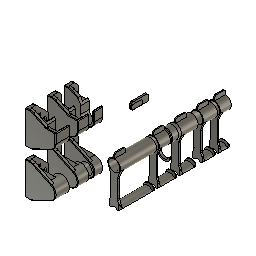
SKADIS_SNS_TapeStorage (Autodesk Fusion 360 design; units mm, degrees)
Autodesk Fusion 360 part; units mm, degrees
(part 1 of 2)
sketch "SlotLayout" plane through (0, 0, 0) normal (1, 0, 0) x (0, 1, 0)
  line L0 (-22.4, 25) -> (-22.4, 15)
  line L1 (82.4, 5) -> (82.4, -5)
  line L2 (-37.6, -5) -> (-37.6, 5)
  line L3 (-80, 5) -> (-80, -5) construction
  line L4 (-97.6, 15) -> (-97.6, 25)
  line L5 (2.4, -5) -> (2.4, 5)
  arc A0 (-77.6, 5) -> (-82.4, 5) centre (-80, 5) ccw
  arc A1 (22.4, 25) -> (17.6, 25) centre (20, 25) ccw
  arc A2 (-97.6, 25) -> (-102.4, 25) centre (-100, 25) ccw
  arc A3 (97.6, 15) -> (102.4, 15) centre (100, 15) ccw
  line L6 (-60, 25) -> (-60, 15) construction
  line L7 (-77.6, -5) -> (-77.6, 5)
  arc A4 (77.6, -5) -> (82.4, -5) centre (80, -5) ccw
  line L8 (-40, 5) -> (-40, -5) construction
  line L9 (-57.6, 15) -> (-57.6, 25)
  line L10 (-62.4, 25) -> (-62.4, 15)
  line L11 (-102.4, 25) -> (-102.4, 15)
  line L12 (97.6, 15) -> (97.6, 25)
  arc A5 (-102.4, 15) -> (-97.6, 15) centre (-100, 15) ccw
  line L13 (20, 25) -> (20, 15) construction
  line L14 (22.4, 25) -> (22.4, 15)
  line L15 (-80, 0) -> (0, 0) construction
  line L16 (62.4, 25) -> (62.4, 15)
  line L17 (42.4, 5) -> (42.4, -5)
  arc A6 (2.5, 5) -> (-2.5, 5) centre (0, 5) ccw
  arc A7 (2.4, 5) -> (-2.4, 5) centre (0, 5) ccw
  line L18 (80, 5) -> (80, -5) construction
  arc A8 (82.4, 5) -> (77.6, 5) centre (80, 5) ccw
  arc A9 (-2.5, -5) -> (2.5, -5) centre (0, -5) ccw
  arc A10 (57.6, 15) -> (62.4, 15) centre (60, 15) ccw
  arc A11 (62.4, 25) -> (57.6, 25) centre (60, 25) ccw
  line L19 (17.6, 15) -> (17.6, 25)
  line L20 (-20, 25) -> (-20, 15) construction
  line L21 (-42.4, 5) -> (-42.4, -5)
  line L22 (60, 25) -> (60, 15) construction
  arc A12 (42.4, 5) -> (37.6, 5) centre (40, 5) ccw
  line L23 (-100, 25) -> (-100, 15) construction
  line L24 (100, 25) -> (100, 15) construction
  arc A13 (-57.6, 25) -> (-62.4, 25) centre (-60, 25) ccw
  arc A14 (37.6, -5) -> (42.4, -5) centre (40, -5) ccw
  line L25 (40, 5) -> (40, -5) construction
  line L26 (-17.6, 15) -> (-17.6, 25)
  arc A15 (-17.6, 25) -> (-22.4, 25) centre (-20, 25) ccw
  line L27 (-82.4, 5) -> (-82.4, -5)
  line L28 (-2.5, 5) -> (-2.5, -5)
  line L29 (-2.4, 5) -> (-2.4, -5)
  line L30 (102.4, 25) -> (102.4, 15)
  arc A16 (17.6, 15) -> (22.4, 15) centre (20, 15) ccw
  arc A17 (-22.4, 15) -> (-17.6, 15) centre (-20, 15) ccw
  line L31 (37.6, -5) -> (37.6, 5)
  line L32 (0, 5) -> (0, -5) construction
  arc A18 (-62.4, 15) -> (-57.6, 15) centre (-60, 15) ccw
  arc A19 (-42.4, -5) -> (-37.6, -5) centre (-40, -5) ccw
  arc A20 (-2.4, -5) -> (2.4, -5) centre (0, -5) ccw
  arc A21 (102.4, 25) -> (97.6, 25) centre (100, 25) ccw
  arc A22 (-82.4, -5) -> (-77.6, -5) centre (-80, -5) ccw
  arc A23 (-37.6, 5) -> (-42.4, 5) centre (-40, 5) ccw
  line L33 (77.6, -5) -> (77.6, 5)
  line L34 (57.6, 15) -> (57.6, 25)
  line L35 (2.5, -5) -> (2.5, 5)
  arc A24 (22.4, -15) -> (17.6, -15) centre (20, -15) ccw
  line L36 (17.6, -15) -> (17.6, -25)
  arc A25 (17.6, -25) -> (22.4, -25) centre (20, -25) ccw
  line L37 (22.4, -25) -> (22.4, -15)
  line L38 (-22.4, -25) -> (-22.4, -15)
  arc A26 (-17.6, -15) -> (-22.4, -15) centre (-20, -15) ccw
  arc A27 (-22.4, -25) -> (-17.6, -25) centre (-20, -25) ccw
  line L39 (-17.6, -15) -> (-17.6, -25)
  line L40 (-62.4, -25) -> (-62.4, -15)
  arc A28 (-57.6, -15) -> (-62.4, -15) centre (-60, -15) ccw
  arc A29 (-62.4, -25) -> (-57.6, -25) centre (-60, -25) ccw
  line L41 (-57.6, -15) -> (-57.6, -25)
  arc A30 (57.6, -25) -> (62.4, -25) centre (60, -25) ccw
  line L42 (62.4, -25) -> (62.4, -15)
  arc A31 (62.4, -15) -> (57.6, -15) centre (60, -15) ccw
  line L43 (57.6, -15) -> (57.6, -25)
  point P0 (-20, 20)
  point P1 (-40, 0)
  dimension "d179_1_1_1" = 0
  dimension "d181_1_1_1" = 0
  dimension "d187_1_1_1" = 10
  constraint tangent L27 A22
  constraint tangent L7 A22
  constraint parallel L7 L27
  constraint tangent A0 L7
  constraint tangent A0 L27
  constraint vertical L3
  constraint tangent L21 A19
  constraint tangent L2 A19
  constraint parallel L2 L21
  constraint tangent L2 A23
  constraint tangent L21 A23
  constraint vertical L8
  constraint tangent L29 A20
  constraint tangent L5 A20
  constraint parallel L5 L29
  constraint tangent L5 A7
  constraint tangent A7 L29
  constraint parallel L2 L32
  constraint midpoint L15.start L3
  constraint midpoint L15.end L32
  constraint horizontal L15
  constraint equal L8 L32
  constraint equal L3 L8
  constraint midpoint P1 L8
  constraint coincident P1 L15
  constraint equal A7 A23
  constraint equal A0 A23
  constraint coincident L15.end origin
  constraint symmetric A0.end L1.start L32
  constraint symmetric L1.end L27.end L32
  constraint symmetric L7.start A4.start L32
  constraint symmetric A8.end A0.start L32
  constraint symmetric A4 L32 A22
  constraint symmetric A0 A8 L32
  constraint symmetric L17.start L21.start L32
  constraint symmetric L17.end L21.end L32
  constraint symmetric A14.start L2.start L32
  constraint symmetric A12.end L2.end L32
  constraint symmetric A14 L32 A19
  constraint symmetric A12 L32 A23
  constraint tangent L0 A17
  constraint tangent L26 A17
  constraint parallel L0 L26
  constraint tangent L26 A15
  constraint tangent L0 A15
  constraint vertical L20
  constraint equal L20 L32
  constraint equal A7 A15
  constraint midpoint P0 L20
  constraint symmetric L0.end L14.end L32
  constraint symmetric L26.end A1.end L32
  constraint symmetric L0.start A1.start L32
  constraint symmetric L26.start L19.start L32
  constraint symmetric A1 A15 L32
  constraint symmetric A16 A17 L32
  constraint symmetric A11.end L9.end L32
  constraint symmetric L16.start L10.start L32
  constraint symmetric A11 A13 L32
  constraint symmetric L16.end L10.end L32
  constraint symmetric A10.start L9.start L32
  constraint symmetric A10 L32 A18
  constraint symmetric L12.end L4.end L32
  constraint symmetric L30.start A2.end L32
  constraint symmetric A2 L32 A21
  constraint symmetric A3.end L11.end L32
  constraint symmetric A3.start L4.start L32
  constraint symmetric A3 A5 L32
  constraint symmetric L0.start L15 L38.start
  constraint symmetric L0.end L15 L38.end
  constraint symmetric A10.start L15 A31.end
  constraint symmetric L16.end L15 L42.end
  constraint symmetric L26.start L15 A26.start
  constraint symmetric L26.end L15 A27.end
  constraint symmetric L19.start L15 A24.end
  constraint symmetric A11.end L15 A30.start
  constraint symmetric L14.end L15 A24.start
  constraint symmetric A1.end L15 L36.end
  constraint symmetric A1.start L15 A25.end
  constraint symmetric L16.start L15 A30.end
  constraint symmetric L10.end L15 L40.end
  constraint symmetric L9.start L15 A28.start
  constraint symmetric L9.end L15 A29.end
  constraint symmetric L10.start L15 L40.start
  constraint symmetric A1 L15 A25
  constraint symmetric L15 A10 A31
  constraint symmetric L15 A11 A30
  constraint symmetric L15 A13 A29
  constraint symmetric L15 A15 A27
  constraint symmetric L15 A16 A24
  constraint symmetric L15 A17 A26
  constraint symmetric L15 A18 A28
  measures "d22" distance of A6.centre A9.centre
  measures "d23" radius of A7
  measures "d4" distance of L8 L32
  measures "d25" distance of L3 L8
  measures "d26" distance of L20.end A6.centre
  measures "d27" distance of P0 L15.end
  measures "d107" radius of A3.end
sketch "PrintKey" plane through (0, 0, 0) normal (1, 0, 0) x (0, 1, 0)
  circle A0 centre (0, 0) radius 1.6
  line L0 (2.6, -6.7) -> (-2.6, -6.7)
  line L1 (-2.6, -6.7) -> (-2.6, 6.7)
  line L2 (-2.6, 6.7) -> (2.6, 6.7)
  line L3 (2.6, 6.7) -> (2.6, -6.7)
  line L4 (0, 6.7) -> (0, -6.7) construction
  line L5 (0, 6.7) -> (0, 23.5939) construction
  line L6 (0, 23.5939) -> (-8.4469, 15.1469) construction
  line L7 (-8.4469, 15.1469) -> (8.4469, 15.1469) construction
  line L8 (8.4469, 15.1469) -> (0, 23.5939) construction
  circle A1 centre (0, 0) radius 3.4
  line L9 (17.4, -6.7) -> (17.4, 6.7)
  line L10 (22.6, -6.7) -> (17.4, -6.7)
  line L11 (22.6, 6.7) -> (22.6, -6.7)
  line L12 (17.4, 6.7) -> (22.6, 6.7)
  circle A2 centre (20, 0) radius 1.6
  circle A3 centre (20, 0) radius 3.4
  line L13 (20, 6.7) -> (20, -6.7) construction
  line L14 (37.4, -6.7) -> (37.4, 6.7)
  line L15 (42.6, -6.7) -> (37.4, -6.7)
  line L16 (42.6, 6.7) -> (42.6, -6.7)
  line L17 (37.4, 6.7) -> (42.6, 6.7)
  circle A4 centre (40, 0) radius 1.6
  circle A5 centre (40, 0) radius 3.4
  line L18 (40, 6.7) -> (40, -6.7) construction
  line L19 (57.4, -6.7) -> (57.4, 6.7)
  line L20 (62.6, -6.7) -> (57.4, -6.7)
  line L21 (62.6, 6.7) -> (62.6, -6.7)
  line L22 (57.4, 6.7) -> (62.6, 6.7)
  circle A6 centre (60, 0) radius 1.6
  circle A7 centre (60, 0) radius 3.4
  line L23 (60, 6.7) -> (60, -6.7) construction
  line L24 (-22.6, -6.7) -> (-22.6, 6.7)
  line L25 (-22.6, 6.7) -> (-17.4, 6.7)
  line L26 (-17.4, -6.7) -> (-22.6, -6.7)
  line L27 (-17.4, 6.7) -> (-17.4, -6.7)
  line L28 (-20, 6.7) -> (-20, -6.7) construction
  circle A8 centre (-20, 0) radius 3.4
  circle A9 centre (-20, 0) radius 1.6
  line L29 (-42.6, -6.7) -> (-42.6, 6.7)
  line L30 (-42.6, 6.7) -> (-37.4, 6.7)
  line L31 (-37.4, -6.7) -> (-42.6, -6.7)
  line L32 (-37.4, 6.7) -> (-37.4, -6.7)
  line L33 (-40, 6.7) -> (-40, -6.7) construction
  circle A10 centre (-40, 0) radius 3.4
  circle A11 centre (-40, 0) radius 1.6
  line L34 (-62.6, -6.7) -> (-62.6, 6.7)
  line L35 (-62.6, 6.7) -> (-57.4, 6.7)
  line L36 (-57.4, -6.7) -> (-62.6, -6.7)
  line L37 (-57.4, 6.7) -> (-57.4, -6.7)
  line L38 (-60, 6.7) -> (-60, -6.7) construction
  circle A12 centre (-60, 0) radius 3.4
  circle A13 centre (-60, 0) radius 1.6
  line L39 (-22.6, 13.3) -> (-22.6, 26.7)
  line L40 (-22.6, 26.7) -> (-17.4, 26.7)
  line L41 (-17.4, 26.7) -> (-17.4, 13.3)
  line L42 (-17.4, 13.3) -> (-22.6, 13.3)
  line L43 (-20, 26.7) -> (-20, 13.3) construction
  circle A14 centre (-20, 20) radius 3.4
  circle A15 centre (-20, 20) radius 1.6
  line L44 (0, 0) -> (-32.4518, 0) construction
  line L45 (-22.6, -26.7) -> (-17.4, -26.7)
  circle A16 centre (-20, -20) radius 1.6
  line L46 (-22.6, -13.3) -> (-22.6, -26.7)
  circle A17 centre (-20, -20) radius 3.4
  line L47 (-20, -26.7) -> (-20, -13.3) construction
  line L48 (-17.4, -26.7) -> (-17.4, -13.3)
  line L49 (-17.4, -13.3) -> (-22.6, -13.3)
  point P0 (20, 0)
  point P1 (20, 0)
  point P2 (20, 0)
  point P3 (40, 0)
  point P4 (40, 0)
  point P5 (40, 0)
  point P6 (60, 0)
  point P7 (60, 0)
  point P8 (60, 0)
  dimension "d21" = 13.4
  dimension "d24" = 5.2
  dimension "d28" = 3.2
  dimension "d34" = 6.8
  dimension "d37" = 20
  dimension "d38" = 0
  dimension "d41" = -20
  dimension "d42" = 0
  dimension "d151" = 0
  dimension "d152" = 20
  constraint horizontal L2
  constraint vertical L3
  constraint horizontal L0
  constraint vertical L1
  constraint midpoint L4.start L2
  constraint midpoint L4.end L0
  constraint midpoint A0.centre L4
  constraint coincident A0.centre A1.centre
  constraint perpendicular L2 L5
  constraint perpendicular L5 L7
  constraint midpoint L5 L7
  constraint perpendicular L6 L8
  constraint perpendicular L28 L44
  constraint symmetric L39.start L44 L46.start
  constraint symmetric L39.end L44 L45.start
  constraint symmetric L40.end L44 L45.end
  constraint symmetric L41.end L44 L48.end
  constraint symmetric L43.start L44 L47.start
  constraint symmetric L43.end L44 L47.end
  constraint symmetric A14 L44 A17
  constraint symmetric A15 L44 A16
  measures "d21" distance of L4.end L4.start
  measures "d24" distance of L1 L3
  measures "d28" diameter of A0
  measures "d34" diameter of A1
sketch "Hanger_Profile" plane through (0, 0, 0) normal (0, 1, 0) x (1, 0, 0)
  line L0 (0, 0) -> (60, 0) construction
  circle A0 centre (60, 0) radius 10.2
  circle A1 centre (60, 0) radius 11.4
  line L1 (60, 0) -> (60, 71.4) construction
  arc A2 (51.3397, 62.3861) -> (68.6603, 62.3861) centre (60, 71.4) ccw
  arc A3 (51.3397, 66.4) -> (68.6603, 66.4) centre (60, 71.4) ccw
  line L2 (51.3397, 66.4) -> (51.3397, 58.4)
  line L3 (51.3397, 58.4) -> (54, 51.091)
  line L4 (54, 51.091) -> (54, 9.6933)
  line L5 (51.3397, 66.4) -> (60, 71.4)
  line L6 (60, 71.4) -> (68.6603, 66.4)
  line L7 (68.6603, 66.4) -> (68.6603, 58.4)
  line L8 (68.6603, 58.4) -> (66, 51.091)
  line L9 (66, 51.091) -> (66, 9.6933)
  circle A4 centre (60, 0) radius 10
  line L10 (59, -11.3561) -> (59, -19.3561)
  line L11 (59, -19.3561) -> (61, -19.3561)
  line L12 (61, -19.3561) -> (61, -11.3561)
  line L13 (60, 0) -> (60, -19.3561) construction
  line L14 (49.333, 4.0218) -> (54, 16.4)
  line L15 (70.667, 4.0218) -> (66, 16.4)
  arc A5 (53.9378, 67.9) -> (66.0622, 67.9) centre (60, 71.4) ccw
  point P0 (60, 11.4)
  point P1 (60, 61.4)
  point P2 (60, 58.9)
  dimension "d53" = 1.2
  dimension "d58" = 2.5
  dimension "d60" = 50
  dimension "d62" = 8
  dimension "d64" = 20
  dimension "d65" = 60
  dimension "d66" = 6
  dimension "d93" = 0.2
  dimension "d94" = 2
  dimension "d95" = 8
  dimension "d97" = 20
  dimension "d107" = 12.5
  dimension "d125" = 5
  dimension "d132" = 60
  dimension "d213" = 3
  constraint coincident L0.start origin
  constraint horizontal L0
  constraint coincident L0.end A0.centre
  constraint concentric A0 A1
  constraint perpendicular L0 L1
  constraint coincident A1 P0
  constraint coincident L1 P0
  constraint coincident P1 A3
  constraint coincident L1 P1
  constraint coincident L1.end A2.centre
  constraint coincident A1 L4.end
  constraint parallel L1 L4
  constraint concentric A2 A3
  constraint coincident L5 A3.start
  constraint parallel L1 L2
  constraint parallel L2 L7
  constraint horizontal L2.end L7.end
  constraint horizontal L3.end L8.end
  constraint parallel L4 L9
  constraint horizontal L4.end L9.end
  constraint coincident A1 L9.end
  constraint concentric A0 A4
  constraint coincident A1 L10.start
  constraint vertical L10
  constraint perpendicular L10 L11
  constraint coincident A1 L12.end
  constraint perpendicular L11 L12
  constraint midpoint L11 L13.end
  constraint vertical L13
  constraint coincident L7 A2.end
  constraint coincident A2 P2
  constraint coincident L2 A2.start
  constraint vertical P1 P2
  constraint horizontal A3.start A3.end
  constraint coincident A1 L14.start
  constraint coincident L4 L14.end
  constraint coincident A1 L15.start
  constraint coincident L9 L15.end
  constraint horizontal L14.end L15.end
  constraint tangent A1 L14
  constraint tangent A1 L15
  constraint coincident L5 A5.start
  constraint horizontal A5.start A5.end
  measures "d53" distance of A0 A1
  measures "d58" distance of P1 P2
  measures "d60" distance of P0 P1
  measures "d62" distance of L2.end A3.start
  measures "d64" angle of L3 L4
  measures "d65" angle of L1 L5
  measures "d66" distance of L1 L4
  measures "d93" distance of A0 A4
  measures "d94" distance of L10.end L11.end
  measures "d95" vertical distance of L12.end L13.end
  measures "d97" diameter of A4
  measures "d107" radius of A2
  measures "d125" vertical distance of P0 L14.end
  measures "d132" distance of L0.start L0.end
  measures "d213" distance of A3.start A5.start
sketch "SideBracket_SideProfile" plane through (0, 0, 0) normal (0, 1, 0) x (1, 0, 0)
  line L0 (0, -30) -> (0, 30)
  arc A0 (40, -14.1) -> (46.09, 12.717) centre (40, 0) ccw
  line L1 (46.09, 12.717) -> (10, 30)
  line L2 (10, 30) -> (0, 30)
  circle A1 centre (40, 0) radius 10.1
  circle A2 centre (40, 0) radius 14.1
  line L3 (10, -30) -> (46.09, -12.717)
  line L4 (5, 30) -> (5, -30)
  line L5 (40, 14.1) -> (5, 14.1)
  line L6 (5, 10.1) -> (49.8387, 10.1)
  line L7 (40, -14.1) -> (5, -14.1)
  line L8 (5, -10.1) -> (49.8387, -10.1)
  line L9 (0, -30) -> (10, -30)
  line L10 (50.1, 0) -> (50.1, -13.5)
  line L11 (54.1, -15.75) -> (54.1, 0)
  line L12 (29.9, 0) -> (29.9, -13.5)
  line L13 (25.9, 0) -> (25.9, -15.75)
  line L14 (52.1207, -17) -> (50.1, -13.5)
  line L15 (52.85, -17) -> (27.15, -17)
  arc A3 (52.85, -17) -> (54.1, -15.75) centre (52.85, -15.75) ccw
  arc A4 (25.9, -15.75) -> (27.15, -17) centre (27.15, -15.75) ccw
  line L16 (27.8793, -17) -> (29.9, -13.5)
  line L17 (27.8793, -17) -> (24.338, -23.1338)
  point P0 (60, 0)
  dimension "d133" = 30
  dimension "d134" = 30
  dimension "d136" = 40
  dimension "d137" = 20.2
  dimension "d140" = 4
  dimension "d174" = 5
  dimension "d175" = 10
  dimension "d178" = 4
  dimension "d182" = 4
  dimension "d183" = 10
  dimension "d184" = 30
  dimension "d258" = 30
  dimension "d259" = 2.5
  dimension "d260" = 17
  dimension "d261" = 30
  dimension "d262" = 3.5
  constraint vertical L0
  constraint coincident L0 origin
  constraint perpendicular L0 L2
  constraint concentric A0 A1
  constraint tangent A0 L1
  constraint concentric A1 A2
  constraint coincident A0.start A2
  constraint coincident A2 L3.end
  constraint tangent A0 L3
  constraint coincident L2 L4.start
  constraint coincident A2 L5.start
  constraint coincident L4 L5.end
  constraint perpendicular L4 L5
  constraint tangent A2 L5
  constraint coincident L4 L6.start
  constraint coincident A2 L6.end
  constraint perpendicular L4 L6
  constraint coincident L4 L7.end
  constraint tangent A2 L7
  constraint perpendicular L4 L7
  constraint coincident L4 L8.start
  constraint coincident A2 L8.end
  constraint perpendicular L4 L8
  constraint perpendicular L0 L9
  constraint coincident A1 L10.start
  constraint vertical L10
  constraint coincident A0 L11.end
  constraint vertical L11
  constraint tangent A1 L10
  constraint coincident A1 L12.start
  constraint coincident A2 L13.start
  constraint perpendicular L8 L13
  constraint tangent A2 L13
  constraint tangent A1 L12
  constraint horizontal L10.end L12.end
  constraint tangent L11 A3
  constraint tangent L13 A4
  constraint equal A3 A4
  constraint tangent L15 A4
  constraint perpendicular L13 L15
  constraint vertical L12
  constraint coincident L15 L14.start
  constraint coincident L15 L16.start
  constraint tangent L15 A3
  constraint tangent A2 L11
  constraint coincident L3 L17.end
  constraint parallel L16 L17
  measures "d133" distance of L0.start origin
  measures "d134" distance of L0.end origin
  measures "d136" distance of L0 A0.centre
  measures "d137" diameter of A1
  measures "d140" distance of A0 A1
  measures "d174" distance of L0 L4
  measures "d175" distance of L0.end L1.end
  measures "d178" distance of L5 L6
  measures "d182" distance of L7 L8
  measures "d183" distance of L0.start L3.start
  measures "d184" vertical distance of L0.start A0.centre
  measures "d258" angle of L11 L14
  measures "d259" diameter of A3
  measures "d260" distance of origin L15
  measures "d261" angle of L12 L16
  measures "d262" distance of L10.end L15
sketch "SideBracket_FrontProfile" plane through (0, 0, 0) normal (1, 0, 0) x (0, 1, 0)
  line L0 (-22.4, 25) -> (-22.4, 15) construction
  arc A0 (-22.4, 15) -> (-17.6, 15) centre (-20, 15) ccw construction
  line L1 (-17.6, 15) -> (-17.6, 25) construction
  arc A1 (-17.6, 25) -> (-22.4, 25) centre (-20, 25) ccw construction
  line L2 (2.5, -5) -> (2.5, 5) construction
  arc A2 (2.5, 5) -> (-2.5, 5) centre (0, 5) ccw construction
  arc A3 (-2.5, -5) -> (2.5, -5) centre (0, -5) ccw construction
  line L3 (-2.5, 5) -> (-2.5, -5) construction
  arc A4 (-22.4, -25) -> (-17.6, -25) centre (-20, -25) ccw construction
  line L4 (-22.4, -25) -> (-22.4, -15) construction
  arc A5 (-17.6, -15) -> (-22.4, -15) centre (-20, -15) ccw construction
  line L5 (-17.6, -15) -> (-17.6, -25) construction
  line L6 (-30, 30) -> (-30, 0)
  line L7 (-30, 0) -> (6, 0)
  line L8 (-30, 30) -> (-16, 30)
  line L9 (-16, 30) -> (6, 8)
  line L10 (6, 8) -> (6, 0)
  line L11 (-24, 30) -> (-24, 0)
  line L12 (-24, -30) -> (-24, 0)
  line L13 (-30, -30) -> (-16, -30)
  line L14 (-16, -30) -> (6, -8)
  line L15 (6, -8) -> (6, 0)
  line L16 (-30, -30) -> (-30, 0)
  line L17 (-16, 30) -> (-16, -30)
  line L18 (-10, 30) -> (-10, -30)
  line L19 (-10, -30) -> (-16, -30)
  line L20 (-16, 30) -> (-10, 30)
  point P0 (-20, 20)
  dimension "d145" = 6
  dimension "d146" = 10
  dimension "d148" = 3
  dimension "d153" = 4
  dimension "d154" = 6
  dimension "d159" = 5
  dimension "d198" = 10
  constraint parallel L1 L6
  constraint horizontal L7
  constraint coincident origin L7
  constraint perpendicular L6 L8
  constraint perpendicular L7 L10
  constraint coincident L8 L11.start
  constraint coincident L7 L11.end
  constraint perpendicular L7 L11
  constraint symmetric L6.start L7 L13.start
  constraint symmetric L6.end L7 L16.end
  constraint symmetric L10.end L7 L15.end
  constraint symmetric L7 L8.end L13.end
  constraint symmetric L7 L9.end L14.end
  constraint symmetric L7 L11.start L12.start
  constraint symmetric L7 L11.end L12.end
  constraint vertical L18
  constraint perpendicular L17 L20
  constraint perpendicular L18 L19
  measures "d145" distance of origin L7.end
  measures "d146" distance of P0 L6
  measures "d148" vertical distance of A2.centre L9.end
  measures "d153" horizontal distance of A1.centre L8.end
  measures "d154" distance of L6 L11
  measures "d159" distance of A1.centre L8
  measures "d198" distance of P0 L18
extrude "Extrude2" add sketch "SideBracket_FrontProfile" along normal blind 5 contours L6 L7 L8 L11 | L7 L12 L13 L16 | L7 L8 L11 L17 | L7 L12 L13 L17 | L7 L9 L17 L18 | L7 L14 L17 L18 | L7 L9 L10 L18 | L7 L14 L15 L18 makes body 1 in component "SideBracket_Heavy_"
extrude "Extrude1" add sketch "SideBracket_SideProfile" along normal blind 5 from surface at -30 contours L0 L2 L4 L9 | L3 L4 L7 L9 L13 L15 A4 L17 | L1 L2 A2 L4 L5 | L4 L7 L8 L13 | A2 L4 L5 L6 | A2 L4 L6 L8 L13 | L7 L8 L12 L13 L16 | L7 L13 L15 A4 L16 | L3 L15 L17 | A0 A2 L6 | A2 L8 L12 L13 | A2 L7 L8 L12 L16 | A0 A2 L3 L7 L15 L16 | A0 A1 A2 L6 L10 | A1 A2 L6 L12 | A2 L8 L12 | A0 A2 L8 | A1 | A1 A2 L8 L12 | A0 A1 A2 L8 L10 bodies 1 in component "SideBracket_Heavy_"
extrude "Extrude3" cut sketch "PrintKey" along normal blind 1.2 contours A0 | L0 L1 L3 A1 | L1 L3 A1 | L1 L2 L3 A1 | L39 L41 L42 A14 | L39 L41 A14 | L39 L40 L41 A14 | A15 | L45 L46 A17 L48 | L46 A17 L48 | L46 A17 L48 L49 | A16 bodies 1 in component "SideBracket_Heavy_"
extrude "Extrude6" add sketch "SideBracket_SideProfile" along normal blind 10 from surface at -25 contours L4 L7 L8 L13 | A2 L4 L5 L6 | L7 L8 L12 L13 L16 | A0 A2 L6 | A2 L7 L8 L12 L16 | A0 A1 A2 L6 L10 | A1 A2 L6 L12 | A0 A2 L8 | A1 A2 L8 L12 | A0 A1 A2 L8 L10 bodies 1 in component "SideBracket_Heavy_"
extrude "Extrude7" add sketch "SideBracket_SideProfile" along normal blind 10 from surface at -15 contours A0 A2 L6 | A0 A1 A2 L6 L10 | A1 A2 L6 L12 | A0 A2 L8 | A1 A2 L8 L12 | A0 A1 A2 L8 L10 bodies 1 in component "SideBracket_Heavy_"
chamfer "Chamfer3" distance 6 angle 45 2 edges at (5, -15, 12.1) (5, -15, -12.1) on bodies 1 in component "SideBracket_Heavy_"
extrude "Extrude4" cut sketch "PrintKey" along normal up to surface (5 mm away) contours A0 | A15 | A16 bodies 1 in component "SideBracket_Heavy_"
extrude "Extrude5" cut sketch "PrintKey" along normal up to surface (2.2 mm away) from surface at 2.8 contours L1 L3 A1 | L3 A1 | L1 A1 | L39 A14 | L39 L41 A14 | L41 A14 | L46 A17 | L46 A17 L48 | A17 L48 bodies 1 in component "SideBracket_Heavy_"
chamfer "Chamfer1" distance 1.8 angle 45 3 edges at (2.8, -23.1699, 18.7705) (2.8, -3.1699, -1.2295) (2.8, -23.1699, -21.2295) on bodies 1 in component "SideBracket_Heavy_"
fillet "Fillet1" radius 4 4 edges at (2.5, -16, 30) (2.5, 6, 8) (2.5, 6, -8) (2.5, -16, -30) on bodies 1 in component "SideBracket_Heavy_"
fillet "Fillet1" radius 16 2 edges at (10, -27.5, -30) (10, -27.5, 30) on bodies 1 in component "SideBracket_Heavy_"
fillet "Fillet1" radius 4 4 edges at (11, -15, 12.1) (11, -15, -12.1) (5, -9, -12.1) (5, -9, 12.1) on bodies 1 in component "SideBracket_Heavy_"
chamfer "Chamfer4" distance 1 angle 45 7 edges at (54.1, -30, 0) (29.6836, -30, 20.5738) (9.9098, -30, 29.6027) (3.1832, -30, 30) (3.1832, -30, -30) (9.9098, -30, -29.6027) (29.6836, -30, -20.5738) on bodies 1 in component "SideBracket_Heavy_"
extrude "Extrude2'" add sketch "SideBracket_FrontProfile" along normal blind 5 separate body contours L6 L7 L8 L11 | L7 L12 L13 L16 | L7 L8 L11 L17 | L7 L12 L13 L17 | L7 L9 L17 L18 | L7 L14 L17 L18 makes body 2 in component "SupportBracket_"
extrude "Extrude1'" add sketch "SideBracket_SideProfile" along normal blind 5 from surface at -30 contours L0 L2 L4 L9 | L3 L4 L7 L9 L13 L15 A4 L17 | L1 L2 A2 L4 L5 | L4 L7 L8 L13 | A2 L4 L5 L6 | A2 L4 L6 L8 L13 | L7 L8 L12 L13 L16 | L7 L13 L15 A4 L16 | L3 L15 L17 | A0 A2 L6 | A2 L8 L12 L13 | A2 L7 L8 L12 L16 | A0 A2 L3 L7 L15 L16 | A0 A1 A2 L6 L10 | A1 A2 L6 L12 | A2 L8 L12 | A0 A2 L8 | A1 A2 L8 L12 | A0 A1 A2 L8 L10 bodies 2 in component "SupportBracket_"
extrude "Extrude3'" cut sketch "PrintKey" along normal blind 1.2 contours A0 | L0 L1 L3 A1 | L1 L3 A1 | L1 L2 L3 A1 | L39 L41 L42 A14 | L39 L41 A14 | L39 L40 L41 A14 | A15 | L45 L46 A17 L48 | L46 A17 L48 | L46 A17 L48 L49 | A16 bodies 2 in component "SupportBracket_"
extrude "Extrude6'" add sketch "SideBracket_SideProfile" along normal blind 10 from surface at -25 contours L4 L7 L8 L13 | A2 L4 L5 L6 | L7 L8 L12 L13 L16 | A0 A2 L6 | A2 L7 L8 L12 L16 | A0 A1 A2 L6 L10 | A1 A2 L6 L12 | A0 A2 L8 | A1 A2 L8 L12 | A0 A1 A2 L8 L10 bodies 2 in component "SupportBracket_"
chamfer "Chamfer3'" distance 5 angle 45 2 edges at (5, -15, 12.1) (5, -15, -12.1) on bodies 2 in component "SupportBracket_"
extrude "Extrude4'" cut sketch "PrintKey" along normal up to surface (5 mm away) contours A0 | A15 | A16 bodies 2 in component "SupportBracket_"
extrude "Extrude5'" cut sketch "PrintKey" along normal up to surface (2.2 mm away) from surface at 2.8 contours L1 L3 A1 | L3 A1 | L1 A1 | L39 A14 | L39 L41 A14 | L41 A14 | L46 A17 | L46 A17 L48 | A17 L48 bodies 2 in component "SupportBracket_"
chamfer "Chamfer1'" distance 1.8 angle 45 2 edges at (2.8, -23.1699, 18.7705) (2.8, -23.1699, -21.2295) on bodies 2 in component "SupportBracket_"
fillet "Fillet2" radius 16 2 edges at (10, -27.5, 30) (10, -27.5, -30) on bodies 2 in component "SupportBracket_"
fillet "Fillet2" radius 4 6 edges at (2.5, -10, -24) (2.5, -16, -30) (2.5, -10, 24) (2.5, -16, 30) (10, -15, 12.1) (10, -15, -12.1) on bodies 2 in component "SupportBracket_"
extrude "Extrude2''" add sketch "SideBracket_FrontProfile" along normal blind 5 separate body contours L6 L7 L8 L11 | L7 L12 L13 L16 | L7 L8 L11 L17 | L7 L12 L13 L17 | L7 L9 L17 L18 | L7 L14 L17 L18 makes body 3 in component "SideBracket_Light_"
extrude "Extrude1''" add sketch "SideBracket_SideProfile" along normal blind 5 from surface at -30 contours L0 L2 L4 L9 | L3 L4 L7 L9 L13 L15 A4 L17 | L1 L2 A2 L4 L5 | L4 L7 L8 L13 | A2 L4 L5 L6 | A2 L4 L6 L8 L13 | L7 L8 L12 L13 L16 | L7 L13 L15 A4 L16 | L3 L15 L17 | A0 A2 L6 | A2 L8 L12 L13 | A2 L7 L8 L12 L16 | A0 A2 L3 L7 L15 L16 | A0 A1 A2 L6 L10 | A1 A2 L6 L12 | A2 L8 L12 | A0 A2 L8 | A1 A2 L8 L12 | A0 A1 A2 L8 L10 bodies 3 in component "SideBracket_Light_"
extrude "Extrude3''" cut sketch "PrintKey" along normal blind 1.2 contours A0 | L0 L1 L3 A1 | L1 L3 A1 | L1 L2 L3 A1 | L39 L41 L42 A14 | L39 L41 A14 | L39 L40 L41 A14 | A15 | L45 L46 A17 L48 | L46 A17 L48 | L46 A17 L48 L49 | A16 bodies 3 in component "SideBracket_Light_"
extrude "Extrude6''" add sketch "SideBracket_SideProfile" along normal blind 10 from surface at -25 contours L4 L7 L8 L13 | A2 L4 L5 L6 | L7 L8 L12 L13 L16 | A0 A2 L6 | A2 L7 L8 L12 L16 | A0 A1 A2 L6 L10 | A1 A2 L6 L12 | A0 A2 L8 | A1 A2 L8 L12 | A0 A1 A2 L8 L10 bodies 3 in component "SideBracket_Light_"
extrude "Extrude8" add sketch "SideBracket_SideProfile" along normal blind 5 from surface at -15 contours A0 A2 L6 | A0 A1 A2 L6 L10 | A1 A2 L6 L12 | A0 A2 L8 | A1 A2 L8 L12 | A0 A1 A2 L8 L10 bodies 3 in component "SideBracket_Light_"
extrude "Extrude9" add sketch "SideBracket_SideProfile" along normal blind 2 from surface at -30 contours A1 bodies 3 in component "SideBracket_Light_"
chamfer "Chamfer3''" distance 5 angle 45 2 edges at (5, -15, 12.1) (5, -15, -12.1) on bodies 3 in component "SideBracket_Light_"
extrude "Extrude4''" cut sketch "PrintKey" along normal up to surface (5 mm away) contours A0 | A15 | A16 bodies 3 in component "SideBracket_Light_"
extrude "Extrude5''" cut sketch "PrintKey" along normal up to surface (2.2 mm away) from surface at 2.8 contours L1 L3 A1 | L3 A1 | L1 A1 | L39 A14 | L39 L41 A14 | L41 A14 | L46 A17 | L46 A17 L48 | A17 L48 bodies 3 in component "SideBracket_Light_"
chamfer "Chamfer1''" distance 1.8 angle 45 2 edges at (2.8, -23.1699, 18.7705) (2.8, -23.1699, -21.2295) on bodies 3 in component "SideBracket_Light_"
fillet "Fillet2'" radius 16 2 edges at (10, -27.5, 30) (10, -27.5, -30) on bodies 3 in component "SideBracket_Light_"
fillet "Fillet2'" radius 4 6 edges at (2.5, -10, -24) (2.5, -16, -30) (2.5, -10, 24) (2.5, -16, 30) (10, -15, 12.1) (10, -15, -12.1) on bodies 3 in component "SideBracket_Light_"
extrude "Extrude1'''" add sketch "Hanger_Profile" along normal blind 3 separate body contours A1 L9 L15 | A1 A2 L2 L3 L4 L7 L8 L9 | A1 L4 L14 | A2 A3 L2 L7 | A3 L5 L6 A5 makes body 4 in component "Hanger_25ID_65W_"
extrude "Extrude2'''" add sketch "Hanger_Profile" along normal blind 60 from surface at 3 contours A3 L5 L6 A5 bodies 4 in component "Hanger_25ID_65W_"
extrude "Extrude3'''" add sketch "Hanger_Profile" along normal blind 1 from surface at 63 contours A2 A3 L2 L7 | A3 L5 L6 A5 bodies 4 in component "Hanger_25ID_65W_"
extrude "Extrude6'''" add sketch "Hanger_Profile" along normal up to surface (65 mm away) contours A1 bodies 4 in component "Hanger_25ID_65W_"
extrude "Extrude7'" add sketch "Hanger_Profile" along normal blind 20 contours A1 L10 L11 L12 bodies 4 in component "Hanger_25ID_65W_"
extrude "Extrude8'" add 1 faces at (58, 3, -27.9637) along direction (0, 1, 0) blind 1 on bodies 4 bodies 4 in component "Hanger_25ID_65W_"
chamfer "Chamfer1'''" distance 2.5 angle 45 6 edges at (60, 0, 19.3561) (60, 20, 19.3561) (60, 63, -61.4) (60, 64, -64.4) (60, 4, -61.4) (60, 4, -11.4) on bodies 4 in component "Hanger_25ID_65W_"
fillet "Fillet5" radius 3 2 edges at (60, 17.5, 19.3561) (60, 2.5, 19.3561) on bodies 4 in component "Hanger_25ID_65W_"
fillet "Fillet5" radius 3 3 edges at (68.6603, 63.5, -62.3861) (51.3397, 63.5, -62.3861) (60, 4, -13.9) on bodies 4 in component "Hanger_25ID_65W_"
fillet "Fillet5" radius 6 6 edges at (51.3397, 2, -58.4) (54, 2, -51.091) (66, 2, -51.091) (68.6603, 2, -58.4) (66, 2, -16.4) (54, 2, -16.4) on bodies 4 in component "Hanger_25ID_65W_"
extrude "Extrude1''''" add sketch "Hanger_Profile" along normal blind 3 separate body contours A1 L9 L15 | A1 A2 L2 L3 L4 L7 L8 L9 | A1 L4 L14 | A2 A3 L2 L7 | A3 L5 L6 A5 makes body 5 in component "Hanger_25ID_35W_"
extrude "Extrude2''''" add sketch "Hanger_Profile" along normal blind 30 from surface at 3 contours A3 L5 L6 A5 bodies 5 in component "Hanger_25ID_35W_"
extrude "Extrude3''''" add sketch "Hanger_Profile" along normal blind 1 from surface at 33 contours A2 A3 L2 L7 | A3 L5 L6 A5 bodies 5 in component "Hanger_25ID_35W_"
extrude "Extrude6''''" add sketch "Hanger_Profile" along normal up to surface (35 mm away) contours A1 bodies 5 in component "Hanger_25ID_35W_"
extrude "Extrude7''" add sketch "Hanger_Profile" along normal blind 20 contours A1 L10 L11 L12 bodies 5 in component "Hanger_25ID_35W_"
chamfer "Chamfer1''''" distance 2.5 angle 45 6 edges at (60, 0, 19.3561) (60, 20, 19.3561) (60, 3, -11.4) (60, 3, -61.4) (60, 33, -61.4) (60, 34, -64.4) on bodies 5 in component "Hanger_25ID_35W_"
fillet "Fillet5'" radius 3 3 edges at (60, 17.5, 19.3561) (60, 2.5, 19.3561) (60, 3, -13.9) on bodies 5 in component "Hanger_25ID_35W_"
fillet "Fillet5'" radius 3 2 edges at (68.6603, 33.5, -62.3861) (51.3397, 33.5, -62.3861) on bodies 5 in component "Hanger_25ID_35W_"
fillet "Fillet5'" radius 6 6 edges at (51.3397, 1.5, -58.4) (54, 1.5, -51.091) (66, 1.5, -51.091) (68.6603, 1.5, -58.4) (66, 1.5, -16.4) (54, 1.5, -16.4) on bodies 5 in component "Hanger_25ID_35W_"
extrude "Extrude1'''''" add sketch "Hanger_Profile" along normal blind 3 separate body contours A1 L9 L15 | A1 A2 L2 L3 L4 L7 L8 L9 | A1 L4 L14 | A2 A3 L2 L7 | A3 L5 L6 A5 makes body 6 in component "Hanger_25ID_30W_"
extrude "Extrude2'''''" add sketch "Hanger_Profile" along normal blind 25 from surface at 3 contours A3 L5 L6 A5 bodies 6 in component "Hanger_25ID_30W_"
extrude "Extrude3'''''" add sketch "Hanger_Profile" along normal blind 1 from surface at 28 contours A2 A3 L2 L7 | A3 L5 L6 A5 bodies 6 in component "Hanger_25ID_30W_"
extrude "Extrude6'''''" add sketch "Hanger_Profile" along normal up to surface (30 mm away) contours A1 bodies 6 in component "Hanger_25ID_30W_"
extrude "Extrude7'''" add sketch "Hanger_Profile" along normal blind 20 contours A1 L10 L11 L12 bodies 6 in component "Hanger_25ID_30W_"
chamfer "Chamfer1'''''" distance 2.5 angle 45 6 edges at (60, 0, 19.3561) (60, 20, 19.3561) (60, 3, -11.4) (60, 3, -61.4) (60, 28, -61.4) (60, 29, -64.4) on bodies 6 in component "Hanger_25ID_30W_"
fillet "Fillet5''" radius 3 3 edges at (60, 17.5, 19.3561) (60, 2.5, 19.3561) (60, 3, -13.9) on bodies 6 in component "Hanger_25ID_30W_"
fillet "Fillet5''" radius 3 2 edges at (68.6603, 28.5, -62.3861) (51.3397, 28.5, -62.3861) on bodies 6 in component "Hanger_25ID_30W_"
fillet "Fillet5''" radius 6 6 edges at (51.3397, 1.5, -58.4) (54, 1.5, -51.091) (66, 1.5, -51.091) (68.6603, 1.5, -58.4) (66, 1.5, -16.4) (54, 1.5, -16.4) on bodies 6 in component "Hanger_25ID_30W_"
extrude "Extrude1''''''" add sketch "Hanger_Profile" along normal blind 3 separate body contours A1 L9 L15 | A1 A2 L2 L3 L4 L7 L8 L9 | A1 L4 L14 | A2 A3 L2 L7 | A3 L5 L6 A5 makes body 7 in component "Hanger_25ID_25W_"
extrude "Extrude2''''''" add sketch "Hanger_Profile" along normal blind 20 from surface at 3 contours A3 L5 L6 A5 bodies 7 in component "Hanger_25ID_25W_"
extrude "Extrude3''''''" add sketch "Hanger_Profile" along normal blind 1 from surface at 23 contours A2 A3 L2 L7 | A3 L5 L6 A5 bodies 7 in component "Hanger_25ID_25W_"
extrude "Extrude6''''''" add sketch "Hanger_Profile" along normal up to surface (25 mm away) contours A1 bodies 7 in component "Hanger_25ID_25W_"
extrude "Extrude7''''" add sketch "Hanger_Profile" along normal blind 20 contours A1 L10 L11 L12 bodies 7 in component "Hanger_25ID_25W_"
chamfer "Chamfer1''''''" distance 2.5 angle 45 6 edges at (60, 0, 19.3561) (60, 20, 19.3561) (60, 3, -11.4) (60, 3, -61.4) (60, 23, -61.4) (60, 24, -64.4) on bodies 7 in component "Hanger_25ID_25W_"
fillet "Fillet5'''" radius 3 3 edges at (60, 17.5, 19.3561) (60, 2.5, 19.3561) (60, 3, -13.9) on bodies 7 in component "Hanger_25ID_25W_"
fillet "Fillet5'''" radius 3 2 edges at (68.6603, 23.5, -62.3861) (51.3397, 23.5, -62.3861) on bodies 7 in component "Hanger_25ID_25W_"
fillet "Fillet5'''" radius 6 6 edges at (51.3397, 1.5, -58.4) (54, 1.5, -51.091) (66, 1.5, -51.091) (68.6603, 1.5, -58.4) (66, 1.5, -16.4) (54, 1.5, -16.4) on bodies 7 in component "Hanger_25ID_25W_"
extrude "Extrude1'''''''" add sketch "Hanger_Profile" along normal blind 3 separate body contours A1 L9 L15 | A1 A2 L2 L3 L4 L7 L8 L9 | A1 L4 L14 | A2 A3 L2 L7 | A3 L5 L6 A5 makes body 8 in component "Hanger_25ID_20W_"
extrude "Extrude2'''''''" add sketch "Hanger_Profile" along normal blind 15 from surface at 3 contours A3 L5 L6 A5 bodies 8 in component "Hanger_25ID_20W_"
extrude "Extrude3'''''''" add sketch "Hanger_Profile" along normal blind 1 from surface at 18 contours A2 A3 L2 L7 | A3 L5 L6 A5 bodies 8 in component "Hanger_25ID_20W_"
extrude "Extrude6'''''''" add sketch "Hanger_Profile" along normal up to surface (20 mm away) contours A1 bodies 8 in component "Hanger_25ID_20W_"
extrude "Extrude7'''''" add sketch "Hanger_Profile" along normal blind 20 contours A1 L10 L11 L12 bodies 8 in component "Hanger_25ID_20W_"
chamfer "Chamfer1'''''''" distance 2.5 angle 45 6 edges at (60, 0, 19.3561) (60, 20, 19.3561) (60, 3, -11.4) (60, 3, -61.4) (60, 18, -61.4) (60, 19, -64.4) on bodies 8 in component "Hanger_25ID_20W_"
fillet "Fillet5''''" radius 3 3 edges at (60, 17.5, 19.3561) (60, 2.5, 19.3561) (60, 3, -13.9) on bodies 8 in component "Hanger_25ID_20W_"
fillet "Fillet5''''" radius 3 2 edges at (68.6603, 18.5, -62.3861) (51.3397, 18.5, -62.3861) on bodies 8 in component "Hanger_25ID_20W_"
fillet "Fillet5''''" radius 6 6 edges at (51.3397, 1.5, -58.4) (54, 1.5, -51.091) (66, 1.5, -51.091) (68.6603, 1.5, -58.4) (66, 1.5, -16.4) (54, 1.5, -16.4) on bodies 8 in component "Hanger_25ID_20W_"
sketch "HangerLabel_Profile" plane through (0, 0, 0) normal (1, 0, 0) x (0, 1, 0)
  line L0 (0, 11.3561) -> (0, 23.7561)
  line L1 (0, 23.7561) -> (30, 23.7561)
  line L2 (30, 23.7561) -> (30, 11.3561)
  line L3 (30, 11.3561) -> (0, 11.3561)
  arc A0 (3.7426, 19.3561) -> (1.6213, 18.4774) centre (3.7426, 16.3561) ccw
  line L4 (1.6213, 18.4774) -> (0, 16.8561)
  line L5 (0, 16.8561) -> (0, 11.3561)
  line L6 (0, 11.3561) -> (20, 11.3561)
  line L7 (20, 11.3561) -> (20, 16.8561)
  line L8 (20, 16.8561) -> (18.3787, 18.4774)
  arc A1 (18.3787, 18.4774) -> (16.2574, 19.3561) centre (16.2574, 16.3561) ccw
  line L9 (16.2574, 19.3561) -> (3.7426, 19.3561)
  line L10 (0, 17.1389) -> (2.4172, 19.5561)
  line L11 (2.4172, 19.5561) -> (17.5828, 19.5561)
  line L12 (17.5828, 19.5561) -> (20.2, 16.9389)
  line L13 (20.2, 16.9389) -> (20.2, 11.3561)
  dimension "d214" = 12.4
  dimension "d215" = 0.2
  dimension "d216" = 0.2
  dimension "d218" = 0.2
  dimension "d219" = 0.2
  dimension "d220" = 30
  constraint vertical L0
  constraint perpendicular L0 L1
  constraint perpendicular L1 L2
  constraint perpendicular L2 L3
  constraint coincident L0.start L3.end
  constraint parallel L4 L10
  constraint perpendicular L0 L11
  constraint coincident L3 L13.end
  constraint perpendicular L3 L13
  constraint parallel L8 L12
  constraint coincident L0 L10.start
  measures "d214" distance of L1 L3
  measures "d215" distance of L7 L13
  measures "d216" distance of L9 L11
  measures "d218" distance of L4 L10
  measures "d219" distance of L8 L12
  measures "d220" distance of L0.end L1.end
extrude "Extrude1''''''''" add sketch "HangerLabel_Profile" along normal blind 1.1 separate body contours L0 L1 L2 L3 L10 L11 L12 L13 makes body 9 in component "HangerLabel_"
extrude "Extrude2''''''''" add sketch "HangerLabel_Profile" along normal blind 0.4 from surface at 1.1 bodies 9 in component "HangerLabel_"
chamfer "Chamfer1''''''''" distance 2 angle 45 2 edges at (0.75, 30, 23.7561) (0.75, 0, 23.7561) on bodies 9 in component "HangerLabel_"
chamfer "Chamfer1''''''''" distance 1 angle 45 2 edges at (0.75, 30, 11.3561) (1.3, 0, 11.3561) on bodies 9 in component "HangerLabel_"
mirror "Mirror1" about plane through (0, 0, 0) normal (-1, 0, 0) of bodies 9 merged in component "HangerLabel_"
move_body "Move1" bodies 3 to x (1, 0, 0) y (0, 1, 0) z (0, 0, 1) at (0, -120, 0) in component "SideBracket_Light_"
move_body "Move1'" bodies 1 to x (1, 0, 0) y (0, 1, 0) z (0, 0, 1) at (0, -160, 0) in component "SideBracket_Heavy_"
move_body "Move1''" bodies 4 to x (1, 0, 0) y (0, 1, 0) z (0, 0, 1) at (0, -90, 0) in component "Hanger_25ID_65W_"
sketch "HangerHook_Profile" plane through (0, 0, 0) normal (0, 1, 0) x (1, 0, 0)
  circle A0 centre (60, 0) radius 11.4
  circle A1 centre (60, 0) radius 10.2
  line L0 (67.3886, 8.6815) -> (54.5558, 19.6031)
  arc A2 (67.8934, 28.873) -> (54.5558, 19.6031) centre (60, 26) ccw
  line L1 (48.6, 0) -> (48.6, 26)
  arc A3 (70.7125, 29.899) -> (48.6, 26) centre (60, 26) ccw
  line L2 (70.7125, 29.899) -> (67.8934, 28.873)
  line L3 (67.8934, 28.873) -> (60, 26) construction
  line L4 (60, 26) -> (60, 0) construction
  dimension "d248" = 3
  dimension "d249" = 26
  dimension "d250" = 110
  constraint coincident A0 L0.start
  constraint tangent L0 A2
  constraint coincident A0 L1.start
  constraint tangent L1 A3
  constraint coincident A2.centre A3.centre
  constraint vertical A0.centre A2.centre
  constraint vertical L1
  constraint collinear L2 L3
  constraint tangent A0 L1
  constraint coincident A0.centre A1.centre
  constraint tangent A0 L0
  measures "d248" distance of A2.start A3.start
  measures "d249" distance of A2.centre A0.centre
  measures "d250" angle of L3 L4
extrude "Extrude1'''''''''" add sketch "HangerHook_Profile" along normal blind 4 separate body makes body 10 in component "Hanger_Hook_20Spacer"
fillet "Fillet1'" radius 1 2 edges at (67.8934, 2, -28.873) (70.7125, 2, -29.899) on bodies 10 in component "Hanger_Hook_20Spacer"
extrude "Extrude1''''''''''" add sketch "HangerHook_Profile" along normal blind 4 separate body makes body 11 in component "Hanger_Hook_Thin"
fillet "Fillet1''" radius 1 2 edges at (67.8934, 2, -28.873) (70.7125, 2, -29.899) on bodies 11 in component "Hanger_Hook_Thin"
extrude "Extrude2'''''''''" add sketch "HangerHook_Profile" along normal blind 20 contours A0 bodies 10 in component "Hanger_Hook_20Spacer"
move_body "Move1'''" bodies 5 to x (1, 0, 0) y (0, 1, 0) z (0, 0, 1) at (0, -20, 0) in component "Hanger_25ID_35W_"
move_body "Move1''''" bodies 6 to x (1, 0, 0) y (0, 1, 0) z (0, 0, 1) at (0, 20, 0) in component "Hanger_25ID_30W_"
move_body "Move1'''''" bodies 7 to x (1, 0, 0) y (0, 1, 0) z (0, 0, 1) at (0, 60, 0) in component "Hanger_25ID_25W_"
move_body "Move1''''''" bodies 8 to x (1, 0, 0) y (0, 1, 0) z (0, 0, 1) at (0, 90, 0) in component "Hanger_25ID_20W_"
chamfer "Chamfer5" distance 1 angle 45 7 edges at (29.6836, -150, 20.5738) (54.1, -150, 0) (29.6836, -150, -20.5738) (9.9098, -150, -29.6027) (3.1832, -150, -30) (3.1832, -150, 30) (9.9098, -150, 29.6027) on bodies 3 in component "SideBracket_Light_"
chamfer "Chamfer5'" distance 1 angle 45 7 edges at (29.6836, -30, 20.5738) (54.1, -30, 0) (29.6836, -30, -20.5738) (9.9098, -30, -29.6027) (3.1832, -30, -30) (3.1832, -30, 30) (9.9098, -30, 29.6027) on bodies 2 in component "SupportBracket_"
extrude "Extrude1'''''''''''" add sketch "Hanger_Profile" along normal blind 2 separate body contours A1 makes body 12 in component "RingSpacer"
extrude "Extrude2''''''''''" add sketch "SideBracket_FrontProfile" along normal blind 5 separate body contours L6 L7 L8 L11 | L7 L12 L13 L16 | L7 L8 L11 L17 | L7 L12 L13 L17 | L7 L9 L17 L18 | L7 L14 L17 L18 | L7 L9 L10 L18 | L7 L14 L15 L18 makes body 13 in component "SideBracket_Heavy_ DropIn"
extrude "Extrude1''''''''''''" add sketch "SideBracket_SideProfile" along normal blind 5 from surface at -30 bodies 13 in component "SideBracket_Heavy_ DropIn"
extrude "Extrude3''''''''" cut sketch "PrintKey" along normal blind 1.2 contours A0 | L0 L1 L3 A1 | L1 L3 A1 | L1 L2 L3 A1 | L39 L41 L42 A14 | L39 L41 A14 | L39 L40 L41 A14 | A15 | L45 L46 A17 L48 | L46 A17 L48 | L46 A17 L48 L49 | A16 bodies 13 in component "SideBracket_Heavy_ DropIn"
extrude "Extrude6''''''''" add sketch "SideBracket_SideProfile" along normal blind 10 from surface at -25 contours L4 L7 L8 L13 | A2 L4 L5 L6 | L7 L8 L12 L13 L16 | L7 L13 L15 A4 L16 | A0 A2 L6 | A2 L8 L12 L13 | A0 A1 A2 L6 L10 | A1 A2 L6 L12 | A0 A2 L10 L11 L14 L15 A3 bodies 13 in component "SideBracket_Heavy_ DropIn"
extrude "Extrude7''''''" add sketch "SideBracket_SideProfile" along normal blind 10 from surface at -15 contours L7 L8 L12 L13 L16 | L7 L13 L15 A4 L16 | A0 A2 L6 | A2 L8 L12 L13 | A0 A1 A2 L6 L10 | A1 A2 L6 L12 | A0 A2 L10 L11 L14 L15 A3 bodies 13 in component "SideBracket_Heavy_ DropIn"
chamfer "Chamfer3'''" distance 6 angle 45 2 edges at (5, -15, 12.1) (5, -15, -12.1) on bodies 13 in component "SideBracket_Heavy_ DropIn"
extrude "Extrude4'''" cut sketch "PrintKey" along normal up to surface (5 mm away) contours A0 | A15 | A16 bodies 13 in component "SideBracket_Heavy_ DropIn"
extrude "Extrude5'''" cut sketch "PrintKey" along normal up to surface (2.2 mm away) from surface at 2.8 contours L1 L3 A1 | L3 A1 | L1 A1 | L39 A14 | L39 L41 A14 | L41 A14 | L46 A17 | L46 A17 L48 | A17 L48 bodies 13 in component "SideBracket_Heavy_ DropIn"
chamfer "Chamfer1'''''''''" distance 1.8 angle 45 3 edges at (2.8, -23.1699, 18.7705) (2.8, -3.1699, -1.2295) (2.8, -23.1699, -21.2295) on bodies 13 in component "SideBracket_Heavy_ DropIn"
fillet "Fillet1'''" radius 4 4 edges at (2.5, -16, 30) (2.5, 6, 8) (2.5, 6, -8) (2.5, -16, -30) on bodies 13 in component "SideBracket_Heavy_ DropIn"
fillet "Fillet1'''" radius 16 2 edges at (10, -27.5, -30) (10, -27.5, 30) on bodies 13 in component "SideBracket_Heavy_ DropIn"
fillet "Fillet1'''" radius 4 5 edges at (11, -15, 12.1) (11, -15, -12.1) (5, -9, -12.1) (5, -9, 12.1) (37.1463, -27.5, 17) on bodies 13 in component "SideBracket_Heavy_ DropIn"
chamfer "Chamfer4'" distance 1 angle 45 10 edges at (51.9306, -30, -7.5147) (54.1, -30, 7.875) (53.7339, -30, 16.6339) (44.9982, -30, 17) (3.1832, -30, -30) (9.9098, -30, -29.6027) (29.6836, -30, -20.5738) (3.1832, -30, 30) (9.9098, -30, 29.6027) (24.8021, -30, 22.9115) on bodies 13 in component "SideBracket_Heavy_ DropIn"
move_body "Move1'''''''" bodies 13 to x (1, 0, 0) y (0, 1, 0) z (0, 0, 1) at (0, -160, 0) in component "SideBracket_Heavy_ DropIn"
extrude "Extrude2'''''''''''" add sketch "SideBracket_FrontProfile" along normal blind 5 separate body contours L6 L7 L8 L11 | L7 L12 L13 L16 | L7 L8 L11 L17 | L7 L12 L13 L17 | L7 L9 L17 L18 | L7 L14 L17 L18 makes body 14 in component "SupportBracket_ DropIn"
extrude "Extrude1'''''''''''''" add sketch "SideBracket_SideProfile" along normal blind 5 from surface at -30 contours L0 L2 L4 L9 | L3 L4 L7 L9 L13 L15 A4 L17 | L1 L2 A2 L4 L5 | L4 L7 L8 L13 | A2 L4 L5 L6 | A2 L4 L6 L8 L13 | L7 L8 L12 L13 L16 | L7 L13 L15 A4 L16 | A0 A2 L6 | A2 L8 L12 L13 | A0 A1 A2 L6 L10 | A1 A2 L6 L12 | A0 A2 L10 L11 L14 L15 A3 bodies 14 in component "SupportBracket_ DropIn"
extrude "Extrude3'''''''''" cut sketch "PrintKey" along normal blind 1.2 contours A0 | L0 L1 L3 A1 | L1 L3 A1 | L1 L2 L3 A1 | L39 L41 L42 A14 | L39 L41 A14 | L39 L40 L41 A14 | A15 | L45 L46 A17 L48 | L46 A17 L48 | L46 A17 L48 L49 | A16 bodies 14 in component "SupportBracket_ DropIn"
extrude "Extrude6'''''''''" add sketch "SideBracket_SideProfile" along normal blind 10 from surface at -25 contours L4 L7 L8 L13 | A2 L4 L5 L6 | L7 L8 L12 L13 L16 | L7 L13 L15 A4 L16 | A0 A2 L6 | A2 L8 L12 L13 | A0 A1 A2 L6 L10 | A1 A2 L6 L12 | A0 A2 L10 L11 L14 L15 A3 bodies 14 in component "SupportBracket_ DropIn"
chamfer "Chamfer3''''" distance 5 angle 45 2 edges at (5, -15, 12.1) (5, -15, -12.1) on bodies 14 in component "SupportBracket_ DropIn"
extrude "Extrude4''''" cut sketch "PrintKey" along normal up to surface (5 mm away) contours A0 | A15 | A16 bodies 14 in component "SupportBracket_ DropIn"
extrude "Extrude5''''" cut sketch "PrintKey" along normal up to surface (2.2 mm away) from surface at 2.8 contours L1 L3 A1 | L3 A1 | L1 A1 | L39 A14 | L39 L41 A14 | L41 A14 | L46 A17 | L46 A17 L48 | A17 L48 bodies 14 in component "SupportBracket_ DropIn"
chamfer "Chamfer1''''''''''" distance 1.8 angle 45 2 edges at (2.8, -23.1699, 18.7705) (2.8, -23.1699, -21.2295) on bodies 14 in component "SupportBracket_ DropIn"
fillet "Fillet2''" radius 16 2 edges at (10, -27.5, 30) (10, -27.5, -30) on bodies 14 in component "SupportBracket_ DropIn"
fillet "Fillet2''" radius 4 6 edges at (2.5, -10, -24) (2.5, -16, -30) (2.5, -10, 24) (2.5, -16, 30) (10, -15, 12.1) (10, -15, -12.1) on bodies 14 in component "SupportBracket_ DropIn"
chamfer "Chamfer5''" distance 1 angle 45 7 edges at (18.8075, -30, 25.7822) (51.9306, -30, -7.5147) (29.6836, -30, -20.5738) (9.9098, -30, -29.6027) (3.1832, -30, -30) (3.1832, -30, 30) (9.9098, -30, 29.6027) on bodies 14 in component "SupportBracket_ DropIn"
extrude "Extrude2''''''''''''" add sketch "SideBracket_FrontProfile" along normal blind 5 separate body contours L6 L7 L8 L11 | L7 L12 L13 L16 | L7 L8 L11 L17 | L7 L12 L13 L17 | L7 L9 L17 L18 | L7 L14 L17 L18 makes body 15 in component "SideBracket_Light_DropIn"
extrude "Extrude1''''''''''''''" add sketch "SideBracket_SideProfile" along normal blind 5 from surface at -30 bodies 15 in component "SideBracket_Light_DropIn"
extrude "Extrude3''''''''''" cut sketch "PrintKey" along normal blind 1.2 contours A0 | L0 L1 L3 A1 | L1 L3 A1 | L1 L2 L3 A1 | L39 L41 L42 A14 | L39 L41 A14 | L39 L40 L41 A14 | A15 | L45 L46 A17 L48 | L46 A17 L48 | L46 A17 L48 L49 | A16 bodies 15 in component "SideBracket_Light_DropIn"
extrude "SlotLayout" add sketch "SideBracket_SideProfile" along normal blind 10 from surface at -25 contours L4 L7 L8 L13 | A2 L4 L5 L6 | L7 L8 L12 L13 L16 | L7 L13 L15 A4 L16 | A0 A2 L6 | A2 L8 L12 L13 | A0 A1 A2 L6 L10 | A1 A2 L6 L12 | A0 A2 L10 L11 L14 L15 A3 bodies 15 in component "SideBracket_Light_DropIn"
extrude "Extrude8''" add sketch "SideBracket_SideProfile" along normal blind 5 from surface at -15 contours L7 L8 L12 L13 L16 | L7 L13 L15 A4 L16 | A0 A2 L6 | A2 L8 L12 L13 | A0 A1 A2 L6 L10 | A1 A2 L6 L12 | A0 A2 L10 L11 L14 L15 A3 bodies 15 in component "SideBracket_Light_DropIn"
extrude "Extrude9'" add sketch "SideBracket_SideProfile" along normal blind 2 from surface at -30 contours A1 bodies 15 in component "SideBracket_Light_DropIn"
chamfer "Chamfer3'''''" distance 5 angle 45 2 edges at (5, -15, 12.1) (5, -15, -12.1) on bodies 15 in component "SideBracket_Light_DropIn"
extrude "Extrude4'''''" cut sketch "PrintKey" along normal up to surface (5 mm away) contours A0 | A15 | A16 bodies 15 in component "SideBracket_Light_DropIn"
extrude "Extrude5'''''" cut sketch "PrintKey" along normal up to surface (2.2 mm away) from surface at 2.8 contours L1 L3 A1 | L3 A1 | L1 A1 | L39 A14 | L39 L41 A14 | L41 A14 | L46 A17 | L46 A17 L48 | A17 L48 bodies 15 in component "SideBracket_Light_DropIn"
chamfer "Chamfer1'''''''''''" distance 1.8 angle 45 2 edges at (2.8, -23.1699, 18.7705) (2.8, -23.1699, -21.2295) on bodies 15 in component "SideBracket_Light_DropIn"